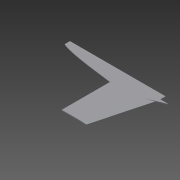
# Autodesk Inventor part: wing
Saved by Autodesk Inventor 2014 SP1 (Build 180222100, 222)
## iProperties
Created: 2018-05-06
Part Number: wing
Material: Generic
Document SubType Name: Modeling
Designer: Dadang
Density: 1 g/cm^3
Appearance: Default
Author: Dadang
Autodesk Inventor part; units mm, degrees
ref_plane "YZ Plane" through (0, 0, 0) normal (1, 0, 0) x (0, 1, 0)
ref_plane "XZ Plane" through (0, 0, 0) normal (0, 1, 0) x (-1, 0, 0)
ref_plane "XY Plane" through (0, 0, 0) normal (0, 0, 1) x (1, 0, 0)
sketch "Sketch1" plane through (0, 0, 0) normal (0, 0, 1) x (1, 0, 0)
  line L0 (0, 0) -> (31.107, -13.144) construction
  line L1 (31.107, -13.144) -> (90.4342, -24.316) construction
  line L2 (90.4342, -24.316) -> (170, -35) construction
  spline S0 degree 3 poles (0, 0) (31.107, -13.144) (90.4342, -24.316) (170, -35) knots 1 1 1 1 2 2 2 2
  line L3 (0, 0) -> (0, 25)
  line L4 (0, 25) -> (458.1698, 25)
  line L5 (263.9103, -47.6101) -> (170, -35)
  line L6 (263.9103, -47.6101) -> (263.9103, -280)
  line L7 (263.9103, -280) -> (383.9103, -280)
  line L8 (458.1698, 25) -> (458.1698, 0)
  line L9 (458.1698, 0) -> (498.1698, 0)
  line L10 (453.2023, -18.73) -> (383.9103, -280)
  line L11 (498.1698, 0) -> (453.2023, -18.73)
  dimension "d5" = 25
  dimension "d21" = 120
  dimension "d22" = 40
  constraints: 18 end point, 3 perpendicular, 3 other
  measures "d5" distance of L0.start L3.end
  measures "d21" distance of L6.end L7.end
  measures "d22" distance of L8.end L9.end
extrude "Extrusion1" add sketch "Sketch1" along normal blind 5
fillet "Fillet1" radius 2.5 2 edges at (66.828, -18.4225, 5) (66.828, -18.4225, 0)
chamfer "Chamfer1" [suppressed]
chamfer "Chamfer2" [suppressed]
fillet "Fillet4" radius 2.5 4 edges at (263.9103, -46.349, 5) (263.9103, -163.8051, 5) (263.9103, -46.349, 0) (263.9103, -163.8051, 0)
chamfer "Chamfer3" distance 30 angle 4 1 edges at (418.5563, -149.365, 5) measured on face at (418.073, -149.2368, 5)
chamfer "Chamfer4" distance 30 angle 4 1 edges at (418.5563, -149.365, 0) measured on face at (418.073, -149.2368, 0)
body "Solid1"
